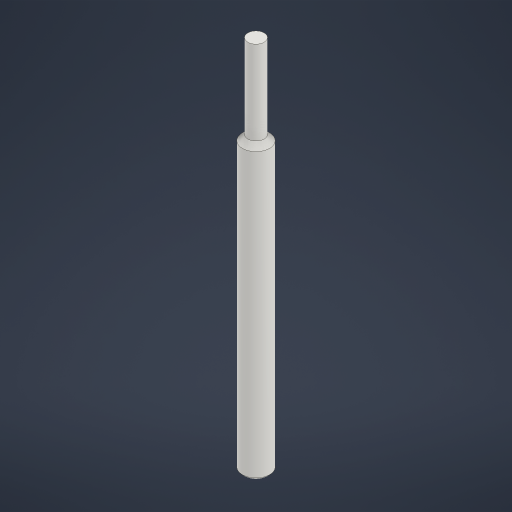
# Autodesk Inventor part: tommybar
Saved by Autodesk Inventor 2023 (Build 270158000, 158)
## iProperties
Created: 2023-03-10
Part Number: tommybar
Material: Steel, High Strength, Low Alloy
Document SubType Name: Modeling
Designer: kamraj
Density: 7.85 g/cm^3
Appearance: Steel
Author: kamraj
Autodesk Inventor part; units mm, degrees
ref_plane "YZ Plane" through (0, 0, 0) normal (1, 0, 0) x (0, 1, 0)
ref_plane "XZ Plane" through (0, 0, 0) normal (0, 1, 0) x (-1, 0, 0)
ref_plane "XY Plane" through (0, 0, 0) normal (0, 0, 1) x (1, 0, 0)
sketch "Sketch1" plane through (0, 0, 0) normal (0, 1, 0) x (-1, 0, 0)
  circle A0 centre (0, 0) radius 10
  dimension "d0" = 20
  constraints: 1 centre point, 1 coincident
  measures "d0" diameter of A0
extrude "Extrusion1" add sketch "Sketch1" against normal blind 213
sketch "Sketch2" plane through (0, 0, 0) normal (0, 1, 0) x (1, 0, 0)
  circle A0 centre (0, 0) radius 6
  dimension "d3" = 12
  constraints: 1 centre point, 1 coincident
  measures "d3" diameter of A0
extrude "Extrusion2" add sketch "Sketch2" along normal blind 62
chamfer "Chamfer1" distance 4 angle 45 1 edges at (10, 0, 0)
sketch "Sketch4" plane through (0, 0, 0) normal (0, 0, 1) x (1, 0, 0)
  line L0 (0, -213) -> (10, -213)
  line L1 (-10, -213) -> (10, -213) projected
  arc A0 (0, -217.8368) -> (10, -213) centre (0, -205.081) ccw
  line L2 (0, -217.8368) -> (0, -213)
  line L3 (0, -213) -> (10, -213)
  point P0 (0, 0)
  point P1 (0, 0)
  point P2 (0, -200.2053)
  constraints: 6 end point, 2 point on circle, 1 centre point, 1 collinear, 1 midpoint
revolve "Revolution1" add sketch "Sketch4" angle 360 mid plane about axis through (0, -217.8368, 0) along (0, 1, 0) fills toward (0.05, -215.4184) open curves L2 A0
body "Solid1"
